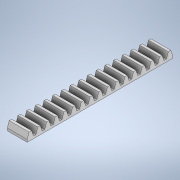
# Autodesk Inventor part: bolt-rack
Saved by Autodesk Inventor 2021 (Build 250183000, 183)
## iProperties
Created: 2024-03-14
Part Number: bolt-rack
Material: Generic
Document SubType Name: Modeling
Designer: 22hamfri
Density: 1 g/cm^3
Appearance: Default
Author: 22hamfri
Autodesk Inventor part; units mm, degrees
ref_plane "YZ Plane" through (0, 0, 0) normal (1, 0, 0) x (0, 1, 0)
ref_plane "XZ Plane" through (0, 0, 0) normal (0, 1, 0) x (-1, 0, 0)
ref_plane "XY Plane" through (0, 0, 0) normal (0, 0, 1) x (1, 0, 0)
sketch "Sketch1" plane through (0, 0, 0) normal (1, 0, 0) x (0, 1, 0)
  line L0 (0, 0) -> (1, 0)
  line L1 (1, 0) -> (3.2, -0.7529)
  line L2 (3.2, -0.7529) -> (3.2, -1.2529)
  line L3 (3.2, -1.2529) -> (0, -1.2529)
  line L4 (0, -1.2529) -> (0, 0)
  line L5 (0, -2.5059) -> (1, -2.5059)
  line L6 (1, -2.5059) -> (3.2, -1.7529)
  line L7 (3.2, -1.7529) -> (3.2, -1.2529)
  line L8 (0, -1.2529) -> (0, -2.5059)
  line L9 (1, -2.5059) -> (1, -3.0059)
  line L10 (1, -3.0059) -> (0, -3.0059)
  line L11 (0, -3.0059) -> (0, -2.5059)
  line L12 (0, -6.0118) -> (1, -6.0118)
  line L13 (1, -6.0118) -> (3.2, -5.2588)
  line L14 (3.2, -5.2588) -> (3.2, -4.7588)
  line L15 (0, -4.7588) -> (0, -6.0118)
  line L16 (3.2, -4.2588) -> (3.2, -4.7588)
  line L17 (1, -3.5059) -> (3.2, -4.2588)
  line L18 (0, -4.7588) -> (0, -3.5059)
  line L19 (1, -3.5059) -> (1, -3.0059)
  line L20 (0, -3.0059) -> (0, -3.5059)
  line L21 (1, -2.5059) -> (1, 0)
  dimension "d1" = 1
  dimension "d2" = 1
  dimension "d3" = 1
  dimension "d4" = 2.2
  dimension "d10" = 3.5059
  constraints: 44 end point, 11 symmetric about line, 5 perpendicular, 2 vertical, 1 horizontal
  measures "d1" distance of L17.start L6.start
  measures "d2" distance of L13.end L16.start
  measures "d3" distance between parallel lines of L20 L19
  measures "d4" distance between parallel lines of L19 L16
  measures "d10" distance of L13.end L7.start
extrude "Extrusion2" add sketch "Sketch1" along normal blind 8 contours L0 L21 L3 L4 | L3 L21 L5 L8 | L5 L9 L10 L11 | L10 L19 L17 L16 L14 L13 L12 L15 L18 L20
extrude "Extrusion3" add sketch "Sketch1" along normal up to surface (8 mm away) contours L1 L2 L3 L21 | L3 L7 L6 L21
pattern_linear "Rectangular Pattern1" count 16 spacing 3.5059 along (0, 0, -1) of "Extrusion2"
equation "\"d15\" = d10"
body "Solid1"
